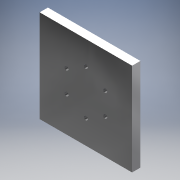
# Autodesk Inventor part: Mounting Plate
Saved by Autodesk Inventor 2019 (Build 230136000, 136)
## iProperties
Created: 2019-08-29
Part Number: Mounting Plate
Material: Aluminum 6061
Document SubType Name: Modeling
Designer: Rick Szalay
Density: 2.7 g/cm^3
Appearance: Aluminum - Flat
Author: Rick Szalay
Autodesk Inventor part; units mm, degrees
ref_plane "YZ Plane" through (0, 0, 0) normal (1, 0, 0) x (0, 1, 0)
ref_plane "XZ Plane" through (0, 0, 0) normal (0, 1, 0) x (-1, 0, 0)
ref_plane "XY Plane" through (0, 0, 0) normal (0, 0, 1) x (1, 0, 0)
sketch "Sketch1" plane through (0, 0, 0) normal (0, 0, 1) x (1, 0, 0)
  line L0 (88.9, -88.9) -> (-88.9, -88.9)
  line L1 (-88.9, -88.9) -> (-88.9, 88.9)
  line L2 (-88.9, 88.9) -> (88.9, 88.9)
  line L3 (88.9, 88.9) -> (88.9, -88.9)
  line L4 (88.9, -88.9) -> (-88.9, 88.9) construction
  line L5 (-88.9, -88.9) -> (88.9, 88.9) construction
  point P0 (0, 0)
  dimension "d2" = 177.8
  constraints: 12 end point, 2 midpoint, 2 parallel, 2 perpendicular, 1 horizontal
  measures "d2" distance of L0.end L1.end
extrude "Extrusion1" add sketch "Sketch1" along normal blind 15.875
sketch "Sketch2" plane through (0, 0, 0) normal (0, 0, -1) x (-1, 0, 0)
  circle A0 centre (0, 0) radius 60.325 projected
  circle A1 centre (0, 42.9196) radius 9.6774 projected
  circle A2 centre (-37.1695, 21.4598) radius 9.6774 projected
  circle A3 centre (-37.1695, -21.4598) radius 9.6774 projected
  circle A4 centre (0, -42.9196) radius 9.6774 projected
  circle A5 centre (37.1695, -21.4598) radius 9.6774 projected
  circle A6 centre (37.1695, 21.4598) radius 9.6774 projected
  line L0 (18.829, -36.4227) -> (14.1966, -28.3993) projected
  arc A7 (-14.1966, -28.3993) -> (14.1966, -28.3993) centre (0, 0) ccw projected
  line L1 (-14.1966, -28.3993) -> (-18.829, -36.4227) projected
  line L2 (-18.829, -36.4227) -> (-22.1285, -34.5177) projected
  line L3 (-22.1285, -34.5177) -> (-17.4962, -26.4943) projected
  arc A8 (-31.6928, -1.905) -> (-17.4962, -26.4943) centre (0, 0) ccw projected
  line L4 (-31.6928, -1.905) -> (-40.9575, -1.905) projected
  line L5 (-40.9575, -1.905) -> (-40.9575, 1.905) projected
  line L6 (-40.9575, 1.905) -> (-31.6928, 1.905) projected
  arc A9 (-17.4962, 26.4943) -> (-31.6928, 1.905) centre (0, 0) ccw projected
  line L7 (-17.4962, 26.4943) -> (-22.1285, 34.5177) projected
  line L8 (-22.1285, 34.5177) -> (-18.829, 36.4227) projected
  line L9 (-18.829, 36.4227) -> (-14.1966, 28.3993) projected
  arc A10 (14.1966, 28.3993) -> (-14.1966, 28.3993) centre (0, 0) ccw projected
  line L10 (14.1966, 28.3993) -> (18.829, 36.4227) projected
  line L11 (18.829, 36.4227) -> (22.1285, 34.5177) projected
  line L12 (22.1285, 34.5177) -> (17.4962, 26.4943) projected
  arc A11 (31.6928, 1.905) -> (17.4962, 26.4943) centre (0, 0) ccw projected
  line L13 (31.6928, 1.905) -> (40.9575, 1.905) projected
  line L14 (40.9575, 1.905) -> (40.9575, -1.905) projected
  line L15 (40.9575, -1.905) -> (31.6928, -1.905) projected
  arc A12 (17.4962, -26.4943) -> (31.6928, -1.905) centre (0, 0) ccw projected
  line L16 (17.4962, -26.4943) -> (22.1285, -34.5177) projected
  line L17 (22.1285, -34.5177) -> (18.829, -36.4227) projected
  point P0 (0, 0)
hole "Hole1" at (0, 42.9196, 0) at (37.1695, 21.4598, 0) at (37.1695, -21.4598, 0) at (0, -42.9196, 0) at (-37.1695, -21.4598, 0) at (-37.1695, 21.4598, 0) direction (0, 0, 1) diameter 7.7978 end through all thread size "3/8-16 UNC" class "2B" standard "ANSI Unified Screw Threads"
sketch "Sketch3" plane through (0, 0, 15.875) normal (0, 0, 1) x (1, 0, 0)
  circle A0 centre (0, 0) radius 20.6375 projected
  point P0 (0, 0)
hole "Hole2" at (0, 0, 15.875) direction (0, 0, -1) diameter 50.8 end through all
body "Solid1"
